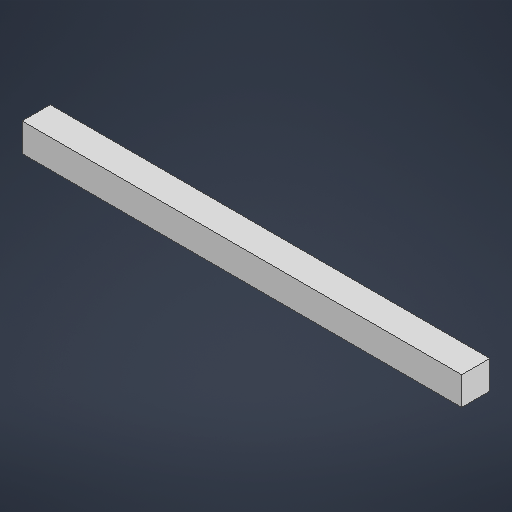
# Autodesk Inventor part: Torsion
Saved by Autodesk Inventor 2025 (Build 290162000, 162)
## iProperties
Created: 2024-12-26
Part Number: Torsion
Material: Типовые
Document SubType Name: Modeling
Designer: khrip
Density: 1 g/cm^3
Appearance: По умолчанию
Author: khrip
Autodesk Inventor part; units mm, degrees
ref_plane "YZ Plane" through (0, 0, 0) normal (1, 0, 0) x (0, 1, 0)
ref_plane "XZ Plane" through (0, 0, 0) normal (0, 1, 0) x (-1, 0, 0)
ref_plane "XY Plane" through (0, 0, 0) normal (0, 0, 1) x (1, 0, 0)
sketch "Эскиз1" plane through (0, 0, 0) normal (1, 0, 0) x (0, 1, 0)
  line L0 (2.25, -2.25) -> (-2.25, -2.25)
  line L1 (-2.25, -2.25) -> (-2.25, 2.25)
  line L2 (-2.25, 2.25) -> (2.25, 2.25)
  line L3 (2.25, 2.25) -> (2.25, -2.25)
  line L4 (2.25, -2.25) -> (-2.25, 2.25) construction
  line L5 (-2.25, -2.25) -> (2.25, 2.25) construction
  point P0 (0, 0)
  dimension "d0" = 4.5
  dimension "d1" = 4.5
  constraints: 12 end point, 2 midpoint, 2 parallel, 1 horizontal, 1 perpendicular
  measures "d0" distance of L1.end L2.end
  measures "d1" distance of L0.end L1.end
extrude "Выдавливание1" add sketch "Эскиз1" along normal blind 70
